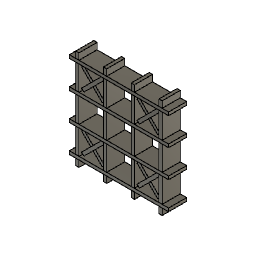
model (Autodesk Fusion 360 design; units mm, degrees)
Autodesk Fusion 360 part; units mm, degrees
sketch "Sketch1" plane through (0, 0, 0) normal (0, 0, 1) x (1, 0, 0) in component "shelf"
  line L0 (0, 0) -> (617.2, 0)
  line L1 (617.2, 0) -> (617.2, 112.5)
  line L2 (617.2, 112.5) -> (0, 112.5)
  line L3 (0, 112.5) -> (0, 0)
  line L4 (40, 112.5) -> (60, 112.5)
  line L5 (60, 112.5) -> (60, 56.25)
  line L6 (60, 56.25) -> (40, 56.25)
  line L7 (40, 56.25) -> (40, 112.5)
  line L8 (232.4, 112.5) -> (232.4, 56.25)
  line L9 (232.4, 56.25) -> (212.4, 56.25)
  line L10 (212.4, 56.25) -> (212.4, 112.5)
  line L11 (212.4, 112.5) -> (232.4, 112.5)
  line L12 (404.8, 112.5) -> (404.8, 56.25)
  line L13 (404.8, 56.25) -> (384.8, 56.25)
  line L14 (384.8, 56.25) -> (384.8, 112.5)
  line L15 (384.8, 112.5) -> (404.8, 112.5)
  line L16 (577.2, 112.5) -> (577.2, 56.25)
  line L17 (577.2, 56.25) -> (557.2, 56.25)
  line L18 (557.2, 56.25) -> (557.2, 112.5)
  line L19 (557.2, 112.5) -> (577.2, 112.5)
  dimension "d5" = 112.5
  dimension "d9" = 617.2
  dimension "d10" = 56.25
  dimension "d11" = 20
  dimension "d12" = 40
  dimension "d15" = 172.4
  dimension "d16" = 0
  constraint horizontal L0
  constraint vertical L1
  constraint horizontal L2
  constraint vertical L3
  constraint coincident L0.start L3.end
  constraint horizontal L4
  constraint vertical L5
  constraint horizontal L6
  constraint vertical L7
  constraint coincident L2 L4.start
  measures "d5" distance of L0.start L2.end
  measures "d9" distance of L0.start L0.end
  measures "d10" distance of L4.start L6.end
  measures "d11" distance of L5.end L6.end
  measures "d12" distance of L3 L7
extrude "Extrude1" add sketch "Sketch1" along normal blind 20 contours L0 L1 L2 L3 L5 L6 L7 L8 L9 L10 L12 L13 L14 L16 L17 L18 makes body 1 in component "shelf"
pattern_linear "R-Pattern1" count 4 spacing 172.4 along (0, 0, 1) of bodies 1 makes body 2 at (283.2, 18.75, 172.4) makes body 3 at (283.2, 18.75, 344.8) makes body 4 at (283.2, 18.75, 517.2) in component "shelf"
copy_body "CopyPasteBodies1" bodies 4 3 2 1 makes body 5 makes body 6 makes body 7 makes body 8 in component "shelf"
copy_body "CopyPasteBodies4" bodies 2 4 8 3 makes body 9 makes body 10 makes body 11 makes body 12 in component "shelf"
move_body "Move4" bodies 9 10 11 12 to x (0, 0, 1) y (0, -1, 0) z (1, 0, 0) at (40, 112.5, -40) in component "shelf"
ref_plane "WorkPlane1" through (212.4, 56.25, 172.4) normal (-0.707107, 0, 0.707107) x (0, -1, 0) in component "crosses"
sketch "Sketch1 (2)" plane through (212.4, 56.25, 172.4) normal (-0.707107, 0, 0.707107) x (0, -1, 0) in component "crosses"
  line L0 (0, 0) -> (56.25, 0) construction
  line L1 (56.25, -215.5261) -> (0, -215.5261) construction
  line L2 (56.25, -215.5261) -> (56.25, 0) construction
  line L3 (-45, -16.5631) -> (45, -16.5631)
  line L4 (45, -16.5631) -> (45, -198.9631)
  line L5 (45, -198.9631) -> (-45, -198.9631)
  line L6 (-45, -198.9631) -> (-45, -16.5631)
  line L7 (15, 0) -> (15, -16.5631) construction
  line L8 (15, -198.9631) -> (15, -215.5261) construction
  line L9 (0, 0) -> (0, -215.5261) construction
  line L10 (0, -107.7631) -> (-45, -107.7631) construction
  line L11 (0, -107.7631) -> (45, -107.7631) construction
  line L12 (-45, -97.7631) -> (0, -97.7631)
  line L13 (0, -97.7631) -> (0, -117.7631)
  line L14 (0, -117.7631) -> (-45, -117.7631)
  line L15 (-45, -117.7631) -> (-45, -97.7631)
  line L16 (-22.5, -107.7631) -> (-22.5, -97.7631) construction
  line L17 (-22.5, -107.7631) -> (-22.5, -117.7631) construction
  point P0 (56.25, -215.5261)
  dimension "d26" = 90
  dimension "d28" = 182.4
  dimension "d33" = 20
  constraint coincident L0.start L9.start
  constraint horizontal L0
  constraint coincident P0 L1.start
  constraint horizontal L1
  constraint vertical L2
  constraint horizontal L3
  constraint vertical L4
  constraint horizontal L5
  constraint vertical L6
  constraint coincident L0 L7.start
  constraint coincident L3 L7.end
  constraint perpendicular L3 L7
  constraint coincident L5 L8.start
  constraint coincident L1 L8.end
  constraint perpendicular L1 L8
  constraint equal L7 L8
  constraint collinear L7 L8
  constraint perpendicular L1 L9
  constraint midpoint L9 L10.start
  constraint midpoint L6 L10.end
  constraint midpoint L4 L11.end
  constraint equal L10 L11
  constraint horizontal L12
  constraint vertical L13
  constraint horizontal L14
  constraint vertical L15
  constraint coincident L9 L13.end
  constraint coincident L6 L12.start
  constraint midpoint L10 L16.start
  constraint midpoint L12 L16.end
  constraint midpoint L14 L17.end
  constraint equal L16 L17
  measures "d26" distance of L4 L6
  measures "d28" distance of L3.end L4.end
  measures "d33" distance of L12 L14
extrude "Extrude1'" add sketch "Sketch1 (2)" along normal blind 10 and the other way blind 10 separate body contours L3 L4 L5 L6 L12 L13 L14 makes body 13 in component "crosses"
copy_body "CopyPasteBodies1'" bodies 13 makes body 14 in component "crosses"
move_body "Move1" bodies 14 to x (1, 0, 0) y (0, -1, 0) z (0, 0, -1) at (0, 112.5, 192.4) in component "crosses"
pattern_linear "R-Pattern1'" count 2 spacing 344.8 along (0, 0, 1) count 2 spacing 344.8 along (1, 0, 0) of bodies 14 13 makes body 15 at (83.7798, 56.25, 402.722) makes body 16 at (519.278, 56.25, 148.6202) makes body 17 at (519.278, 56.25, 493.4202) makes body 18 at (83.7798, 56.25, 479.278) makes body 19 at (519.278, 56.25, 43.7798) makes body 20 at (519.278, 56.25, 388.5798) in component "crosses"
component "shelf" placed x (1, 0, 0) y (0, 1, 0) z (0, 0, 1) at (0, 0, 0)
component "crosses" placed x (1, 0, 0) y (0, 1, 0) z (0, 0, 1) at (0, 0, 0)
equation "squareSize = 6 in"
equation "materialThickness = 20 mm"
equation "squareMaterialWidth = 112.5 mm"
equation "crossMaterialWidth = 90 mm"
equation "d5 = squareMaterialWidth"
equation "squareOverhang = 40 mm"
equation "squareCount = 3"
equation "squareMemberLength = 2 * squareOverhang + squareCount * squareSize + ( squareCount + 1 ) * materialThickness"
equation "d9 = squareMemberLength"
equation "d10 = d5 / 2"
equation "d11 = materialThickness"
equation "d12 = squareOverhang"
equation "d13 = squareCount + 1"
equation "d15 = squareSize + materialThickness"
equation "squareSpacing = squareSize + materialThickness"
equation "d18 = materialThickness"
equation "d20 = squareCount + 1"
equation "d22 = squareSpacing"
equation "crossLength = squareSize + 30 mm"
equation "d26 = crossMaterialWidth"
equation "d28 = crossLength"
equation "d29 = materialThickness / 2"
equation "d31 = materialThickness / 2"
equation "d33 = materialThickness"
equation "d34 = crossCount"
equation "d35 = crossCount"
equation "d36 = 2 * squareSpacing"
equation "d37 = 2 * squareSpacing"
equation "crossCount = ceil(squareCount / 2)"
